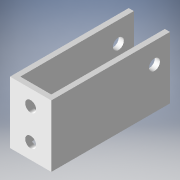
# Autodesk Inventor part: 15102898-16-P-0311
Saved by Autodesk Inventor 2017 (Build 210142000, 142)
## iProperties
Created: 2016-11-06
Part Number: 15102898-16-P-0311
Material: Generic
Document SubType Name: Modeling
Designer: gus
Mass: 17.0562 g
Surface Area: 118.562 cm^2
Volume: 17.0562 cm^3
Density: 1 g/cm^3
Appearance: Default
Author: gus
Autodesk Inventor part; units mm, degrees
ref_plane "YZ Plane" through (0, 0, 0) normal (1, 0, 0) x (0, 1, 0)
ref_plane "XZ Plane" through (0, 0, 0) normal (0, 1, 0) x (-1, 0, 0)
ref_plane "XY Plane" through (0, 0, 0) normal (0, 0, 1) x (1, 0, 0)
sketch "Sketch1" plane through (0, 0, 0) normal (0, 1, 0) x (-1, 0, 0)
  line L0 (0, 0) -> (0, -73.025)
  line L1 (0, -73.025) -> (-3.175, -73.025)
  line L2 (-3.175, -73.025) -> (-3.175, -3.175)
  line L3 (-3.175, -3.175) -> (-22.225, -3.175)
  line L4 (-22.225, -3.175) -> (-22.225, -73.025)
  line L5 (-22.225, -73.025) -> (-25.4, -73.025)
  line L6 (-25.4, -73.025) -> (-25.4, 0)
  line L7 (-25.4, 0) -> (0, 0)
  dimension "d0" = 3.175
  dimension "d1" = 73.025
  dimension "d2" = 3.175
  dimension "d3" = 25.4
  dimension "d4" = 3.175
  constraints: 16 end point, 6 perpendicular, 2 point on line, 1 vertical
  measures "d0" distance of L4.end L5.end
  measures "d1" distance of L5.end L6.end
  measures "d2" distance between parallel lines of L7 L3
  measures "d3" distance of L6.end L0.start
  measures "d4" distance between parallel lines of L0 L2
extrude "Extrusion1" add sketch "Sketch1" along normal blind 38.1
sketch "Sketch2" plane through (25.4, 0, 0) normal (1, 0, 0) x (0, 0, -1)
  line L0 (73.025, 0) -> (73.025, 38.1) projected
  line L1 (73.025, 0) -> (0, 0) projected
  point P0 (63.5, 25.4)
  dimension "d7" = 9.525
  dimension "d8" = 25.4
  measures "d7" distance from line of L0 point (63.5, 25.4)
  measures "d8" distance from line of L1 point (63.5, 25.4)
hole "Hole1" at (25.4, 25.4, -63.5) direction (-1, 0, 0) diameter 6.7469 end through all
sketch "Sketch3" plane through (22.225, 0, -3.175) normal (0, 0, -1) x (-1, 0, 0)
  line L0 (-3.175, 0) -> (22.225, 0) projected
  line L1 (0, 38.1) -> (19.05, 38.1) projected
  line L2 (22.225, 0) -> (22.225, 38.1) projected
  line L3 (-3.175, 0) -> (-3.175, 38.1) projected
  point P0 (9.525, 9.525)
  point P1 (9.525, 28.575)
  point P2 (22.225, 31.75)
  point P3 (-3.175, 31.75)
  dimension "d19" = 9.525
  dimension "d20" = 9.525
  dimension "d21" = 12.7
  dimension "d22" = 12.7
  measures "d19" distance from line of L0 point (9.525, 9.525)
  measures "d20" distance from line of L1 point (9.525, 28.575)
  measures "d21" distance from line of L2 point (9.525, 9.525)
  measures "d22" distance from line of L3 point (9.525, 28.575)
hole "Hole2" at (12.7, 9.525, -3.175) at (12.7, 28.575, -3.175) direction (0, 0, 1) diameter 6.7469 end through all
body "Solid1"
